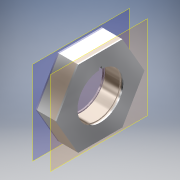
# Autodesk Inventor part: Stopper Outer
Saved by Autodesk Inventor 2019.4 (Build 234330000, 330)
## iProperties
Created: 2020-03-11
Part Number: Stopper Outer
Material: Aluminum 6061
Document SubType Name: Modeling
Designer: Mark
Mass: 43.3087 g
Surface Area: 58.5839 cm^2
Volume: 16.0403 cm^3
Density: 2.7 g/cm^3
Appearance: Aluminum - Flat
Author: Mark
Autodesk Inventor part; units mm, degrees
ref_plane "YZ Plane" through (0, 0, 0) normal (1, 0, 0) x (0, 1, 0)
ref_plane "XZ Plane" through (0, 0, 0) normal (0, 1, 0) x (-1, 0, 0)
ref_plane "XY Plane" through (0, 0, 0) normal (0, 0, 1) x (1, 0, 0)
sketch "Sketch1" plane through (0, 0, 0) normal (1, 0, 0) x (0, 1, 0)
  circle A0 centre (0, 0) radius 15
  line L0 (25, -14.4338) -> (0, -28.8675)
  line L1 (0, -28.8675) -> (-25, -14.4338)
  line L2 (-25, -14.4338) -> (-25, 14.4338)
  line L3 (-25, 14.4338) -> (0, 28.8675)
  line L4 (0, 28.8675) -> (25, 14.4338)
  line L5 (25, 14.4338) -> (25, -14.4338)
  line L6 (0, 0) -> (25, 0)
  line L7 (0, 0) -> (25, 0) construction
  dimension "d0" = 30
  dimension "d1" = 25
  dimension "d2" = 25
  dimension "d3" = 0
  dimension "d4" = 90
  constraints: 16 end point, 2 coincident, 2 horizontal, 1 centre point, 1 collinear, 13 other
  measures "d0" diameter of A0
  measures "d1" distance from line of point (0, 0) L5
  measures "d2" distance of L6.start L6.end
  measures "d3" distance between parallel lines of L6 L7
  measures "d4" angle of L5 L6
extrude "Extrusion1" add sketch "Sketch1" along normal blind 13.6
ref_plane "Work Plane1" through (0.95, 0, 0) normal (-1, 0, 0) x (0, 0, 1)
sketch "Sketch2" plane through (0.95, 0, 0) normal (-1, 0, 0) x (0, 0, 1)
  circle A0 centre (0, 0) radius 15.7
  circle A1 centre (0, 0) radius 10
  dimension "d8" = 31.4
  dimension "d9" = 20
  constraints: 2 centre point, 2 coincident
  measures "d8" diameter of A0
  measures "d9" diameter of A1
extrude "Extrusion2" cut sketch "Sketch2" against normal blind 1.3
ref_plane "Work Plane2" through (12.65, 0, 0) normal (1, 0, 0) x (0, 0, -1)
sketch "Sketch3" plane through (12.65, 0, 0) normal (1, 0, 0) x (0, 0, -1)
  circle A0 centre (0, 0) radius 15.7
  circle A1 centre (0, 0) radius 10
  dimension "d13" = 31.4
  dimension "d14" = 20
  constraints: 2 centre point, 2 coincident
  measures "d13" diameter of A0
  measures "d14" diameter of A1
extrude "Extrusion3" cut sketch "Sketch3" against normal blind 1.3
sketch "Sketch4" plane through (13.6, 0, 0) normal (1, 0, 0) x (0, 0, -1)
  line L0 (-1, 13.6) -> (1, 13.6)
  line L1 (1, 13.6) -> (1, 16.4)
  line L2 (1, 16.4) -> (-1, 16.4)
  line L3 (-1, 16.4) -> (-1, 13.6)
  circle A0 centre (0, 0) radius 15 projected
  line L4 (-1, 13.6) -> (1, 16.4) construction
  line L5 (1, 13.6) -> (-1, 16.4) construction
  line L6 (0, 0) -> (0, 2) construction
  line L7 (0, 0) -> (2, 0) construction
  point P0 (0, 15)
  point P1 (0, 15)
  dimension "d17" = 2
  dimension "d18" = 2.8
  dimension "d19" = 2
  dimension "d20" = 90
  constraints: 16 end point, 3 midpoint, 2 horizontal, 2 parallel, 2 perpendicular, 1 point on line, 1 vertical, 1 vertical alignment, 1 other
  measures "d17" distance of L2.end L1.end
  measures "d18" distance of L1.end L0.end
  measures "d19" distance of L6.start L6.end
  measures "d20" angle of L7 L6
extrude "Extrusion4" cut sketch "Sketch4" against normal blind 32.2 contours L3 A0 L1 L0 | L3 L2 L1 A0 picked at (0.1112, 14.0654)
body "Solid1"
